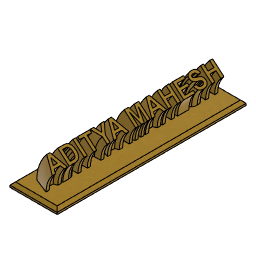
Aditya Nameplate v2 (Autodesk Fusion 360 design; units mm, degrees)
Autodesk Fusion 360 part; units mm, degrees
box "BoxPrimitive1" add length 200 width 50 height 5 placed x (0, 1, 0) y (-1, 0, 0) z (0, 0, 1) at (0, 0, 0)
sketch "Sketch2" plane through (0, 0, 5) normal (0, 0, 1) x (-1, 0, 0)
  line L0 (0, -200) -> (50, -200)
  line L1 (50, -200) -> (50, 0)
  line L2 (50, 0) -> (0, 0)
  line L3 (0, 0) -> (0, -200)
  line L4 (9.5649, -5.6521) -> (9.5649, -195.6521) construction
  line L5 (9.5649, -195.6521) -> (49.5649, -195.6521) construction
  line L6 (49.5649, -195.6521) -> (49.5649, -5.6521) construction
  line L7 (49.5649, -5.6521) -> (9.5649, -5.6521) construction
  dimension "d6" = 16
  text T0 "ADITYA MAHESH" font "Arial" height 16 bold align centre middle in box 190 x 40 at (9.5649, -5.6521) x (0, -1) y (1, 0) spacing 1 kerned
sketch "Sketch4" plane through (0, 0, 0) normal (0, -1, 0) x (1, 0, 0)
  line L0 (-50, 5) -> (-50, 0)
  line L1 (-50, 0) -> (0, 0)
  line L2 (0, 0) -> (0, 5)
  line L3 (0, 5) -> (-50, 5)
  arc A0 (4, 11) -> (0, 5) centre (6.5, 5) ccw
  constraint tangent L2 A0
  constraint coincident L2.end L3.start
sweep "Sweep1" add profiles "Sketch2" path "Sketch4" along A0 for 0.6 of its length starting at (4, 0, 11) heading (-0.9231, 0, -0.3846) section 1 text T0
chamfer "Chamfer1" distance 3 angle 45 4 edges at (-25, 0, 5) (0, 100, 5) (-50, 100, 5) (-25, 200, 5)
